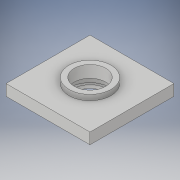
# Autodesk Inventor part: Part2
Saved by Autodesk Inventor 2018 (Build 220112000, 112)
## iProperties
Created: 2018-07-29
Part Number: Part2
Material: Generic
Document SubType Name: Modeling
Designer: BB-8
Density: 1 g/cm^3
Appearance: Default
Author: BB-8
Autodesk Inventor part; units mm, degrees
ref_plane "YZ Plane" through (0, 0, 0) normal (1, 0, 0) x (0, 1, 0)
ref_plane "XZ Plane" through (0, 0, 0) normal (0, 1, 0) x (-1, 0, 0)
ref_plane "XY Plane" through (0, 0, 0) normal (0, 0, 1) x (1, 0, 0)
sketch "Sketch1" plane through (0, 0, 0) normal (0, 1, 0) x (-1, 0, 0)
  line L0 (0, 0) -> (76, 0)
  line L1 (76, 0) -> (76, -76)
  line L2 (76, -76) -> (0, -76)
  line L3 (0, -76) -> (0, 0)
  dimension "d0" = 76
  dimension "d1" = 76
  constraints: 8 end point, 2 parallel, 1 horizontal, 1 perpendicular
  measures "d0" distance of L1.end L2.end
  measures "d1" distance of L0.end L1.end
extrude "Extrusion1" add sketch "Sketch1" along normal blind 10
sketch "Sketch2" plane through (0, 10, 0) normal (0, 1, 0) x (1, 0, 0)
  circle A0 centre (-38, 38) radius 19
  point P0 (0, 0)
  dimension "d4" = 38
  constraints: 1 centre point
  measures "d4" diameter of A0
extrude "Extrusion2" add sketch "Sketch2" along normal blind 4.9
sketch "Sketch8" plane through (0, 0, 0) normal (0, -1, 0) x (1, 0, 0)
  circle A0 centre (-38, -38) radius 27
  point P0 (0, 0)
  dimension "d18" = 54
  constraints: 1 centre point
  measures "d18" diameter of A0
extrude "Extrusion6" add sketch "Sketch8" along normal blind 5
sketch "Sketch9" plane through (-38, -5, -38) normal (0, -1, 0) x (1, 0, 0)
  circle A0 centre (0, 0) radius 15.75
  point P0 (38, 38)
  dimension "d21" = 31.5
  constraints: 1 centre point
  measures "d21" diameter of A0
extrude "Extrusion7" cut sketch "Sketch9" against normal blind 3
sketch "Sketch10" plane through (-38, -2, -38) normal (0, -1, 0) x (1, 0, 0)
  circle A0 centre (0, 0) radius 18
  point P0 (38, 38)
  dimension "d24" = 36
  constraints: 1 centre point
  measures "d24" diameter of A0
extrude "Extrusion8" cut sketch "Sketch10" against normal blind 6.1
sketch "Sketch11" plane through (-38, 14.9, -38) normal (0, 1, 0) x (1, 0, 0)
  circle A0 centre (0, 0) radius 15.75 projected
  circle A1 centre (0, 0) radius 14.25
  point P0 (38, -38)
  dimension "d27" = 28.5
  constraints: 1 centre point, 1 coincident
  measures "d27" diameter of A1
extrude "Extrusion9" cut sketch "Sketch11" against normal blind 10.8 contours A1
body "Solid1"
